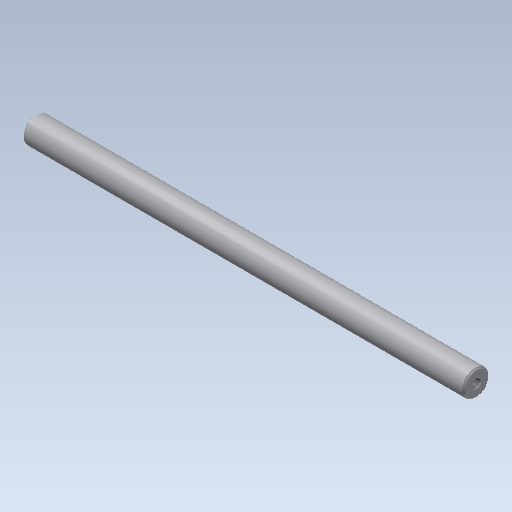
# Autodesk Inventor part: AETTF8-135-M3-N3
Saved by Autodesk Inventor 2020 (Build 240168000, 168)
## iProperties
Created: 2016-05-25
Part Number: AETTF8-135-M3-N3
Catalog Web Link: www.cadenas.de
Description: NETF, ETKF, PETF, SETF, AETTF-Circular Posts - Both Ends Tapped - Thread Diameter Configurable
Vendor: MISUMI
Document SubType Name: Modeling
Designer: psAdmin
Manufacturer: MISUMI
Mass: 18.755 g
Surface Area: 36.0538 cm^2
Volume: 6.69822 cm^3
Density: 2.8 g/cm^3
Material: アルミニウム 2014-T4
Appearance: サテン
Category: PARTsolutions
Company: MISUMI
PSOL_IDENT_0: {$CADENAS_DATA\23d-libs\misumi\metric\19_posts_stands\petf.prj},232 {VTYP=3D},{NB=AETTF8-135-M3-N3},
PSOL_IDENT_1: {LINA=AETTF8-135-M3-N3},{NN=NETF, ETKF, PETF, SETF, AETTF},{DATE=18.11.2015 05:09:36},{GEOMDATE=30.1
PSOL_IDENT_2: 0.2015 07:35:48},{VERSION=},{LINEID=60},{LINESUBID=-1},{WBVAR=MAT,ST,M,N,ALT1,L,ALT2,HL,ALT4,ALT5}
PSOL_IDENT_3: {NB=AETTF8-135-M3-N3},{LINA=AETTF8-135-M3-N3},{KT=DUMMY},{PN=AETTF8-135-M3-N3},{TYPE=AETTF},{MAT=A20
PSOL_IDENT_4: 17},{MATALG= 'LCS','Low Carbon Steel', 'SUS304', 'SUS304', 'A2017', '2017 Aluminum Alloy' },{ST=CA},
PSOL_IDENT_5: {STALG= 'CA', 'Clear Anodize' },{D=8},{M=3.0},{M1=[3,4,5]},{MPITCH=0.500},{MDEPT=9.0},{MAV=3},{N=3.0
PSOL_IDENT_6: },{N1=[3,4,5]},{NPITCH=0.500},{NDEPT=9.0},{NAV=4},{ALT1=},{L=135.0},{LALG=[15:200/0.5]},{LMIN=15.0},
PSOL_IDENT_7: {LMIN1=15},{LMIN2=13},{LMIN21=130},{LMIN22=150},{LMIN23=150},{LMIN3=15},{LMAX=200},{ALT2=},{ALT2ALG=
PSOL_IDENT_8: '', 'w/o HL (Through Hole for Hex Wrench)', '-HL', 'with HL (Through Hole for Hex Wrench)' },{ALT2P
PSOL_IDENT_9: N=},{HL=0},{HLALG=0},{HLMIN=7},{HLMAX=128},{DD=0.0},{DD1=2.5},{ALT4=},{ALT4ALG='','w/o MD (Left End
PSOL_IDENT_10: Change The Effective Tap Depth)','MD','with MD (Left End Change The Effective Tap Depth)'},{ALT4PN=-
PSOL_IDENT_11: M3},{ALT5=},{ALT5ALG='','w/o ND (Right End Change The Effective Tap Depth)','ND','with ND (Right End
PSOL_IDENT_12: Change The Effective Tap Depth)'},{ALT5PN=-N3}
NN: NETF, ETKF, PETF, SETF, AETTF
NT: Circular Posts - Both Ends Tapped - Thread Diameter Configurable
NB: AETTF8-135-M3-N3
NBSYN: $PN.
LINA: AETTF8-135-M3-N3
PN: AETTF8-135-M3-N3
MAT: 2017 Aluminum Alloy
ST: Clear Anodize
D: 8
M: 3.0
N: 3.0
ALT1: w/o LKC (L Dimension Tolerance)
L: 135.0
ALT2: w/o HL (Through Hole for Hex Wrench)
HL: 0
DD: 0.0
ALT4: w/o MD (Left End Change The Effective Tap Depth)
ALT5: w/o ND (Right End Change The Effective Tap Depth)
SUPPLIER: MISUMI
ARTICLENO: AETTF8-135-M3-N3
BOMINFO: AETTF8-135-M3-N3
CREATOR: CADENAS GmbH
Title: AETTF8-135-M3-N3
Author: Cadenas PARTsolutions
Comments: Circular Posts - Both Ends Tapped - Thread Diameter Configurable
Autodesk Inventor part; units mm, degrees
ref_plane "YZ Plane" through (0, 0, 0) normal (1, 0, 0) x (0, 1, 0)
ref_plane "XZ Plane" through (0, 0, 0) normal (0, 1, 0) x (-1, 0, 0)
ref_plane "XY Plane" through (0, 0, 0) normal (0, 0, 1) x (1, 0, 0)
sketch "Sketch_1" plane through (0, 0, 0) normal (0, 0, 1) x (1, 0, 0)
  line L0 (135, 0) -> (0, 0)
  line L1 (0, 0) -> (0, 3.5)
  line L2 (0, 3.5) -> (0.5, 4)
  line L3 (0.5, 4) -> (134.5, 4)
  line L4 (134.5, 4) -> (135, 3.5)
  line L5 (135, 3.5) -> (135, 0)
  line L6 (135, 0) -> (0, 0)
  constraints: 14 end point
revolve "Revolution1" add sketch "Sketch_1" angle 360 about axis through (135, 0, 0) along (1, 0, 0)
sketch "Sketch2" plane through (0, 0, 0) normal (-1, 0, 0) x (0, 0, 1)
  point P0 (0, 0)
hole "Hole1" at (0, 0, 0) direction (1, 0, 0) diameter 2.459 depth 8.2901 tip angle 120 countersink diameter 3 countersink angle 90 thread size "M3x0.5" class "6H" standard "ISO Metric profile"
sketch "Sketch3" plane through (135, 0, 0) normal (1, 0, 0) x (0, 0, -1)
  point P0 (0, 0)
hole "Hole2" at (135, 0, 0) direction (-1, 0, 0) diameter 2.459 depth 8.2901 tip angle 120 countersink diameter 3 countersink angle 90 thread size "M3x0.5" class "6H" standard "ISO Metric profile"
body "Solid1"
